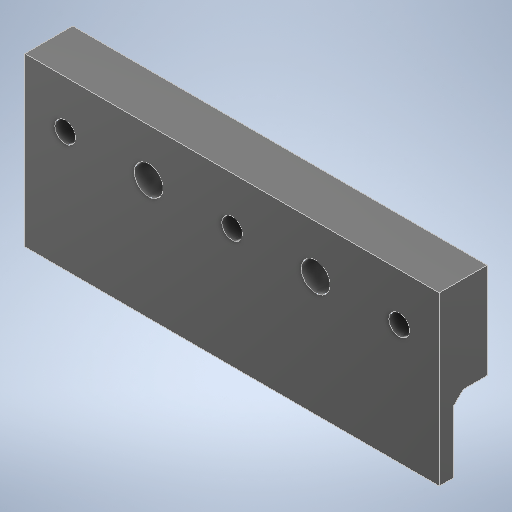
# Autodesk Inventor part: IR_Mount_Plate_1
Saved by Autodesk Inventor 2025.1 (Build 291241020, 241B)
## iProperties
Created: 2024-11-14
Part Number: IR_Mount_Plate_1
Material: PC/ABS Plastic
Document SubType Name: Modeling
Designer: leon-
Density: 1.1 g/cm^3
Appearance: Smooth - Black
Author: leon-
## iProperties of the stored document IR_Mount_Plate_3DPrint.ipt
Created: 2024-11-19
Part Number: IR_Mount_Plate_3DPrint
Material: Generic
Document SubType Name: Modeling
Designer: leon-
Density: 1 g/cm^3
Appearance: Default
Author: leon-
Autodesk Inventor part; units mm, degrees
ref_plane "YZ Plane" through (0, 0, 0) normal (1, 0, 0) x (0, 1, 0)
sketch "Sketch1" plane through (0, 0, 0) normal (0, 0, 1) x (1, 0, 0)
  line L0 (0, 0) -> (260, 0)
  line L1 (260, 0) -> (260, 20)
  line L2 (260, 20) -> (0, 20)
  line L3 (0, 20) -> (0, 0)
  dimension "d0" = 260
  dimension "d1" = 20
  constraints: 8 end point, 2 parallel, 1 horizontal, 1 perpendicular
  measures "d0" distance of L1.end L2.end
  measures "d1" distance of L0.end L1.end
extrude "Extrusion1" add sketch "Sketch1" along normal blind 3
sketch "Sketch2" plane through (0, 0, 0) normal (0, 0, -1) x (-1, 0, 0)
  line L0 (0, 0) -> (-260, 0) projected
  line L1 (-12.5251, -24.7625) -> (-37.9251, -24.7625) projected
  line L2 (-260, 20) -> (0, 20) projected
  point P0 (-25.2251, 30)
  dimension "d5" = 25.4
  dimension "d6" = 12.7
  dimension "d62" = 10
  measures "d5" distance of L1.start L1.end
  measures "d6" horizontal distance of L1.start point (-25.225, 30)
  measures "d62" distance from line of L2 point (-25.225, 30)
sketch "Sketch5" plane through (0, 0, 0) normal (-1, 0, 0) x (0, 0, 1)
  line L0 (0, 20) -> (3, 20) projected
  line L1 (3, 20) -> (-7, 20)
  line L2 (-7, 20) -> (-7, 40)
  line L3 (-7, 40) -> (3, 40)
  line L4 (3, 40) -> (3, 20)
  point P0 (0, 0)
  point P1 (3, 30)
  point P2 (1.5, 20)
  dimension "d31" = 10
  dimension "d32" = 20
  constraints: 8 end point, 2 midpoint, 2 parallel, 1 horizontal, 1 perpendicular
  measures "d31" distance from line of L2 point (3, 30)
  measures "d32" distance from line of point (1.5, 20) L3
extrude "Extrusion3" add sketch "Sketch5" against normal up to surface (260 mm away)
sketch "Sketch6" plane through (0, 0, 3) normal (0, 0, 1) x (1, 0, 0)
  line L0 (0, 0) -> (0, 40) projected
  line L1 (260, 0) -> (260, 40) projected
  line L2 (0, 40) -> (260, 40) projected
  point P0 (42.6875, 30)
  point P1 (77.6125, 30)
  point P2 (182.3875, 30)
  point P3 (217.3125, 30)
  point P4 (112.5375, 30)
  point P5 (147.4625, 30)
  dimension "d35" = 42.6875
  dimension "d46" = 42.6875
  dimension "d47" = 34.925
  dimension "d48" = 34.925
  dimension "d49" = 34.925
  dimension "d50" = 34.925
  dimension "d51" = 10
  constraints: 5 horizontal alignment
  measures "d35" distance from line of point (42.687, 30) L0
  measures "d46" distance from line of L1 point (217.312, 30)
  measures "d47" distance of point (77.612, 30) point (42.687, 30)
  measures "d48" distance of point (217.312, 30) point (182.387, 30)
  measures "d49" distance of point (182.387, 30) point (147.463, 30)
  measures "d50" distance of point (77.612, 30) point (112.537, 30)
  measures "d51" distance from line of L2 point (42.687, 30)
hole "Hole2" at (42.6875, 30, 3) at (77.6125, 30, 3) at (182.3875, 30, 3) at (217.3125, 30, 3) at (112.5375, 30, 3) at (147.4625, 30, 3) direction (0, 0, -1) diameter 6 end through all
hole "Hole3" at (25.2251, 30, 0) direction (0, 0, 1) diameter 4.3 depth 6
pattern_linear "Rectangular Pattern2" count 7 spacing 34.925 along (1, 0, 0) of "Hole3"
chamfer "Chamfer1" distance 2 angle 45 1 edges at (130, 20, 0)
sketch "Sketch7" plane through (0, 0, 0) normal (-1, 0, 0) x (0, 0, 1)
  line L0 (0, 0) -> (3, 0) projected
  line L1 (0, 0) -> (3.6796, 0)
  line L2 (3.6796, 0) -> (3.6796, 5)
  line L3 (3.6796, 5) -> (0, 5)
  line L4 (0, 5) -> (0, 0)
  dimension "d66" = 5
  constraints: 8 end point, 2 parallel, 1 horizontal, 1 perpendicular
  measures "d66" distance of L1.end L2.end
extrude "Extrusion4" cut sketch "Sketch7" against normal through all
ref_plane "Work Plane1" through (173.3333, 20, -7) normal (1, 0, 0) x (0, 0, -1)
ref_plane "Work Plane2" through (86.6667, 20, -7) normal (1, 0, 0) x (0, 0, -1)
sketch "Sketch8" plane through (173.3333, 20, -7) normal (1, 0, 0) x (0, 0, -1)
  line L0 (-10, -15) -> (-7, -15) projected
  line L1 (-7, -15) -> (-7, -2) projected
  line L2 (-5, 0) -> (-7, -2) projected
  line L3 (0, 0) -> (-5, 0) projected
  line L4 (0, 20) -> (0, 0) projected
  line L5 (-10, 20) -> (0, 20) projected
  line L6 (-10, -15) -> (-10, 20) projected
  point P0 (-7, -20)
extrude "Extrusion5" cut sketch "Sketch8" along normal through all
sketch "Sketch9" plane through (86.6667, 20, -7) normal (1, 0, 0) x (0, 0, -1)
  line L0 (0, 13) -> (-10, 13) projected
  line L1 (-7, -15) -> (-10, -15) projected
  line L2 (-7, -2) -> (-7, -15) projected
  line L3 (-5, 0) -> (-7, -2) projected
  line L4 (0, 0) -> (-5, 0) projected
  line L5 (0, 20) -> (0, 0) projected
  line L6 (-10, 20) -> (0, 20) projected
  line L7 (-10, -15) -> (-10, 20) projected
  point P0 (-7, -20)
extrude "Extrusion6" cut sketch "Sketch9" against normal through all
equation "\"d6\" = 0.5 * d5"
equation "\"d46\" = d35"
equation "\"d48\" = d47"
equation "\"d49\" = d47"
equation "\"d50\" = d47"
body "Solid1"
